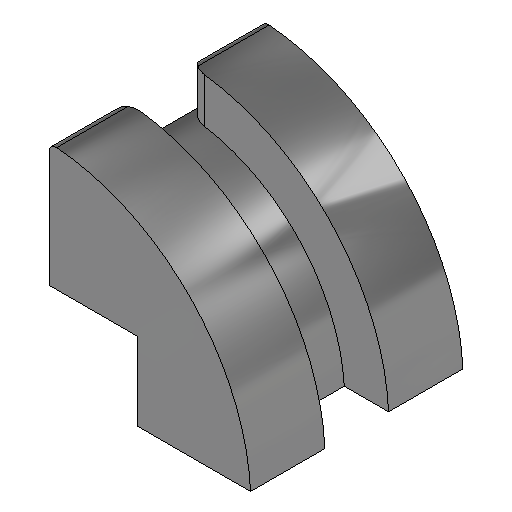
# Autodesk Inventor part: TL20240901-10320CV-020
Saved by Autodesk Inventor 2022.5 (Build 265521000, 521)
## iProperties
Category: FOLLOWER UNIT ASSY
Company: 현대 트랜시스
Created: 2023-04-10
Part Number: TL20240901-10320CV-020
Checked By: 김형민
Engr Approved By: 김형민
User Status: 2 x6
Material: S45C
Description: 0
Document SubType Name: Modeling
Mfg Approved By: 호상태
Designer: 박성규
Stock Number: 020
Density: 7.87 g/cm^3
Appearance: Plating Chrome
Project: MEa-PJT 2LINE
DETAIL: Coveryor Assembly
M/C TITLE: CJ 제일제당 협동로봇 포장시스탬 PILOT 장비
PARTS NAME: Bracket
SPECIFICATION: TA20221101-CV200000-015
DocNumber: 221118_Standard_v1
Folder: .\
VDS_Category: 엔지니어링
Detail Description: Processed products
Title: CHAIN SUPPORTER
Subject: MEa차종 시트조립2라인
Author: 박성규
Revision Number: A
Autodesk Inventor part; units mm, degrees
ref_plane "YZ Plane" through (0, 0, 0) normal (1, 0, 0) x (0, 1, 0)
ref_plane "XZ Plane" through (0, 0, 0) normal (0, 1, 0) x (-1, 0, 0)
sketch "Sketch15" plane through (0, 0, 0) normal (0, 0, 1) x (1, 0, 0)
  circle A0 centre (0, 0) radius 60
  dimension "d88" = 120
  constraints: 1 centre point, 1 coincident
  measures "d88" diameter of A0
extrude "Extrusion7" add sketch "Sketch15" along normal mid plane 60
ref_plane "Work Plane1" through (0, 0, 0) normal (0, 0, 1) x (1, 0, 0)
sketch "Sketch16" plane through (0, 0, 0) normal (0, 0, 1) x (1, 0, 0)
  circle A0 centre (0, 0) radius 60 projected
  circle A1 centre (0, 0) radius 47.5
  dimension "d117" = 95
  constraints: 1 centre point
  measures "d117" diameter of A1
extrude "Extrusion8" cut sketch "Sketch16" along normal mid plane 18
sketch "Sketch17" plane through (0, 0, 0) normal (0, 0, 1) x (1, 0, 0)
  circle A0 centre (0, 0) radius 60 projected
  line L0 (3, 3) -> (59.925, 3)
  line L1 (3, 3) -> (3, 59.925)
  line L2 (28, 25) -> (0, 25)
  line L3 (0, 25) -> (0, 0)
  line L4 (0, 0) -> (28, 0)
  line L5 (28, 0) -> (28, 25)
  point P0 (28, 3)
  point P1 (3, 25)
  dimension "d118" = 3
  dimension "d119" = 3
  dimension "d120" = 22
  dimension "d121" = 25
  constraints: 12 end point, 2 horizontal, 2 parallel, 2 point on circle, 1 perpendicular, 1 vertical
  measures "d118" distance from line of L0 point (0, 0)
  measures "d119" distance from line of L1 point (0, 0)
  measures "d120" distance between parallel lines of L2 L0
  measures "d121" distance between parallel lines of L1 L5
extrude "Extrusion9" cut sketch "Sketch17" along normal through all both and the other way through all contours A0 L1 L2 L3 L4 L5 L0 | L5 L4 L3 L2 L1 L0 | L0 L1 L2 L5
sketch "Sketch19" plane through (3, 25, 30) normal (0, -1, 0) x (1, 0, 0)
  line L0 (0, -60) -> (0, 0) projected
  point P0 (-3, -30)
  point P1 (12.5, -15)
  point P2 (12.5, -45)
  point P3 (0, -30)
  point P4 (12.5, -30)
  point P5 (0, -30)
  dimension "d122" = 30
  dimension "d123" = 15
  dimension "d124" = 12.5
  constraints: 2 midpoint, 2 vertical alignment, 1 horizontal alignment
  measures "d122" distance of point (12.5, -45) point (12.5, -15)
  measures "d123" vertical distance of point (0, -30) point (12.5, -15)
  measures "d124" distance from line of point (12.5, -15) L0
hole "Hole6" at (15.5, 25, 15) at (15.5, 25, -15) at (15.5, 25, 0) direction (0, 1, 0) diameter 4.917 depth 17.1 tip angle 118 thread size "M6x1" class "6H" standard "TS profile"
fillet "Fillet4" radius 2 2 edges at (3, 59.925, -19.5) (3, 59.925, 19.5)
fillet "Fillet5" radius 5 2 edges at (3, 52.5946, -9) (3, 52.5946, 9)
equation "\"d123\" = 0.5 * d122"
body "Solid4"
